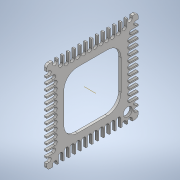
# Autodesk Inventor part: FrontPanelSquishything
Saved by Autodesk Inventor 2020 (Build 240168000, 168)
## iProperties
Created: 2019-07-06
Part Number: FrontPanelSquishything
Material: Generic
Document SubType Name: Modeling
Designer: DDeGo
Density: 1 g/cm^3
Appearance: Default
Author: DDeGo
Autodesk Inventor part; units mm, degrees
ref_plane "YZ Plane" through (0, 0, 0) normal (1, 0, 0) x (0, 1, 0)
ref_plane "XZ Plane" through (0, 0, 0) normal (0, 1, 0) x (-1, 0, 0)
ref_plane "XY Plane" through (0, 0, 0) normal (0, 0, 1) x (1, 0, 0)
sketch "Sketch1" plane through (0, 0, 0) normal (1, 0, 0) x (0, 1, 0)
  line L0 (-78.25, 91.75) -> (78.25, 91.75) construction
  line L1 (91.75, 78.25) -> (91.75, -78.25) construction
  line L2 (78.25, -91.75) -> (-78.25, -91.75) construction
  line L3 (-91.75, -78.25) -> (-91.75, 78.25) construction
  arc A0 (91.75, 78.25) -> (78.25, 91.75) centre (78.25, 78.25) ccw construction
  arc A1 (78.25, -91.75) -> (91.75, -78.25) centre (78.25, -78.25) ccw construction
  arc A2 (-91.75, -78.25) -> (-78.25, -91.75) centre (-78.25, -78.25) ccw construction
  arc A3 (-78.25, 91.75) -> (-91.75, 78.25) centre (-78.25, 78.25) ccw construction
  line L4 (-51.75, 56.75) -> (51.75, 56.75) construction
  line L5 (56.75, 51.75) -> (56.75, -51.75) construction
  line L6 (51.75, -56.75) -> (-51.75, -56.75) construction
  line L7 (-56.75, -51.75) -> (-56.75, 51.75) construction
  arc A4 (-51.75, 56.75) -> (-56.75, 51.75) centre (-51.75, 51.75) ccw construction
  arc A5 (-56.75, -51.75) -> (-51.75, -56.75) centre (-51.75, -51.75) ccw construction
  arc A6 (51.75, -56.75) -> (56.75, -51.75) centre (51.75, -51.75) ccw construction
  arc A7 (56.75, 51.75) -> (51.75, 56.75) centre (51.75, 51.75) ccw construction
  line L8 (78.25, 83.75) -> (-78.25, 83.75)
  arc A8 (-78.25, 83.75) -> (-83.75, 78.25) centre (-78.25, 78.25) ccw
  line L9 (-83.75, 78.25) -> (-83.75, -78.25)
  arc A9 (-83.75, -78.25) -> (-78.25, -83.75) centre (-78.25, -78.25) ccw
  line L10 (-78.25, -83.75) -> (78.25, -83.75)
  arc A10 (78.25, -83.75) -> (83.75, -78.25) centre (78.25, -78.25) ccw
  line L11 (83.75, -78.25) -> (83.75, 78.25)
  arc A11 (83.75, 78.25) -> (78.25, 83.75) centre (78.25, 78.25) ccw
  line L12 (-47.7, 83.75) -> (-47.7, 68.75) construction
  line L13 (-51.75, 83.75) -> (-51.75, 68.75)
  line L14 (-43.65, 68.75) -> (-43.65, 83.75)
  arc A12 (-43.65, 83.75) -> (-51.75, 83.75) centre (-47.7, 83.75) ccw
  arc A13 (-51.75, 68.75) -> (-43.65, 68.75) centre (-47.7, 68.75) ccw
  line L15 (-33.05, 68.75) -> (-33.05, 83.75)
  line L16 (-37.1, 83.75) -> (-37.1, 68.75) construction
  arc A14 (-41.15, 68.75) -> (-33.05, 68.75) centre (-37.1, 68.75) ccw
  arc A15 (-33.05, 83.75) -> (-41.15, 83.75) centre (-37.1, 83.75) ccw
  line L17 (-41.15, 83.75) -> (-41.15, 68.75)
  line L18 (-22.45, 68.75) -> (-22.45, 83.75)
  line L19 (-26.5, 83.75) -> (-26.5, 68.75) construction
  arc A16 (-30.55, 68.75) -> (-22.45, 68.75) centre (-26.5, 68.75) ccw
  arc A17 (-22.45, 83.75) -> (-30.55, 83.75) centre (-26.5, 83.75) ccw
  line L20 (-30.55, 83.75) -> (-30.55, 68.75)
  line L21 (-11.85, 68.75) -> (-11.85, 83.75)
  line L22 (-15.9, 83.75) -> (-15.9, 68.75) construction
  arc A18 (-19.95, 68.75) -> (-11.85, 68.75) centre (-15.9, 68.75) ccw
  arc A19 (-11.85, 83.75) -> (-19.95, 83.75) centre (-15.9, 83.75) ccw
  line L23 (-19.95, 83.75) -> (-19.95, 68.75)
  line L24 (-1.25, 68.75) -> (-1.25, 83.75)
  line L25 (-5.3, 83.75) -> (-5.3, 68.75) construction
  arc A20 (-9.35, 68.75) -> (-1.25, 68.75) centre (-5.3, 68.75) ccw
  arc A21 (-1.25, 83.75) -> (-9.35, 83.75) centre (-5.3, 83.75) ccw
  line L26 (-9.35, 83.75) -> (-9.35, 68.75)
  line L27 (9.35, 68.75) -> (9.35, 83.75)
  line L28 (5.3, 83.75) -> (5.3, 68.75) construction
  arc A22 (1.25, 68.75) -> (9.35, 68.75) centre (5.3, 68.75) ccw
  arc A23 (9.35, 83.75) -> (1.25, 83.75) centre (5.3, 83.75) ccw
  line L29 (1.25, 83.75) -> (1.25, 68.75)
  line L30 (19.95, 68.75) -> (19.95, 83.75)
  line L31 (15.9, 83.75) -> (15.9, 68.75) construction
  arc A24 (11.85, 68.75) -> (19.95, 68.75) centre (15.9, 68.75) ccw
  arc A25 (19.95, 83.75) -> (11.85, 83.75) centre (15.9, 83.75) ccw
  line L32 (11.85, 83.75) -> (11.85, 68.75)
  line L33 (30.55, 68.75) -> (30.55, 83.75)
  line L34 (26.5, 83.75) -> (26.5, 68.75) construction
  arc A26 (22.45, 68.75) -> (30.55, 68.75) centre (26.5, 68.75) ccw
  arc A27 (30.55, 83.75) -> (22.45, 83.75) centre (26.5, 83.75) ccw
  line L35 (22.45, 83.75) -> (22.45, 68.75)
  line L36 (41.15, 68.75) -> (41.15, 83.75)
  line L37 (37.1, 83.75) -> (37.1, 68.75) construction
  arc A28 (33.05, 68.75) -> (41.15, 68.75) centre (37.1, 68.75) ccw
  arc A29 (41.15, 83.75) -> (33.05, 83.75) centre (37.1, 83.75) ccw
  line L38 (33.05, 83.75) -> (33.05, 68.75)
  line L39 (51.75, 68.75) -> (51.75, 83.75)
  line L40 (47.7, 83.75) -> (47.7, 68.75) construction
  arc A30 (43.65, 68.75) -> (51.75, 68.75) centre (47.7, 68.75) ccw
  arc A31 (51.75, 83.75) -> (43.65, 83.75) centre (47.7, 83.75) ccw
  line L41 (43.65, 83.75) -> (43.65, 68.75)
  line L42 (-51.75, 51.75) -> (51.75, -51.75) construction
  line L43 (-58.3, 83.75) -> (-58.3, 71.75) construction
  line L44 (-62.35, 83.75) -> (-62.35, 71.75)
  line L45 (-54.25, 71.75) -> (-54.25, 83.75)
  arc A32 (-54.25, 83.75) -> (-62.35, 83.75) centre (-58.3, 83.75) ccw
  arc A33 (-62.35, 71.75) -> (-54.25, 71.75) centre (-58.3, 71.75) ccw
  line L46 (58.3, 83.75) -> (58.3, 71.75) construction
  line L47 (54.25, 83.75) -> (54.25, 71.75)
  line L48 (62.35, 71.75) -> (62.35, 83.75)
  arc A34 (62.35, 83.75) -> (54.25, 83.75) centre (58.3, 83.75) ccw
  arc A35 (54.25, 71.75) -> (62.35, 71.75) centre (58.3, 71.75) ccw
  line L49 (-68.9, 83.75) -> (-68.9, 79.75) construction
  line L50 (-72.95, 83.75) -> (-72.95, 79.75)
  line L51 (-64.85, 79.75) -> (-64.85, 83.75)
  arc A36 (-64.85, 83.75) -> (-72.95, 83.75) centre (-68.9, 83.75) ccw
  arc A37 (-72.95, 79.75) -> (-64.85, 79.75) centre (-68.9, 79.75) ccw
  line L52 (68.9, 83.75) -> (68.9, 79.75) construction
  line L53 (64.85, 83.75) -> (64.85, 79.75)
  line L54 (72.95, 79.75) -> (72.95, 83.75)
  arc A38 (72.95, 83.75) -> (64.85, 83.75) centre (68.9, 83.75) ccw
  arc A39 (64.85, 79.75) -> (72.95, 79.75) centre (68.9, 79.75) ccw
  point P0 (-47.7, 76.25)
  point P1 (-37.1, 76.25)
  point P2 (-26.5, 76.25)
  point P3 (-15.9, 76.25)
  point P4 (-5.3, 76.25)
  point P5 (5.3, 76.25)
  point P6 (15.9, 76.25)
  point P7 (26.5, 76.25)
  point P8 (37.1, 76.25)
  point P9 (47.7, 76.25)
  point P10 (0, 0)
  point P11 (-58.3, 77.75)
  point P12 (58.3, 77.75)
  point P13 (-68.9, 81.75)
  point P14 (68.9, 81.75)
  dimension "d0" = 13.5
  dimension "d1" = 183.5
  dimension "d2" = 183.5
  dimension "d15" = 35
  dimension "d16" = 35
  dimension "d17" = 35
  dimension "d18" = 35
  dimension "d19" = 5
  dimension "d20" = 8
  dimension "d21" = 15
  dimension "d25" = 10.6
  dimension "d30" = 32
  dimension "d38" = 32
  dimension "d40" = 10.6
  dimension "d41" = 12
  dimension "d42" = 10.6
  dimension "d63" = 4
  dimension "d64" = 4
  dimension "d65" = 10.6
  dimension "d66" = 10.6
  dimension "d67" = 2.5
  constraints: 138 end point, 80 point on circle, 40 centre point, 36 tangent, 12 parallel, 10 equal radius, 8 perpendicular, 6 midpoint, 5 point on line, 3 horizontal, 116 other
  measures "d0" radius of A0
  measures "d1" distance between parallel lines of L2 L0
  measures "d2" distance between parallel lines of L1 L3
  measures "d15" distance between parallel lines of L3 L7
  measures "d16" distance between parallel lines of L0 L4
  measures "d17" distance between parallel lines of L1 L5
  measures "d18" distance between parallel lines of L2 L6
  measures "d19" radius of A4
  measures "d20" distance between parallel lines of L0 L8
  measures "d21" distance of L12.start L12.end
  measures "d25" distance of L14.start L15.start
  measures "d30" distance between parallel lines of L9 L13
  measures "d38" distance between parallel lines of L11 L39
  measures "d40" distance between parallel lines of L44 L13
  measures "d41" distance of L43.start L43.end
  measures "d42" distance between parallel lines of L48 L39
  measures "d63" distance of L49.start L49.end
  measures "d64" distance of L52.start L52.end
  measures "d65" distance between parallel lines of L48 L54
  measures "d66" distance between parallel lines of L50 L44
  measures "d67" distance between parallel lines of L17 L14
extrude "Extrusion1" add sketch "Sketch1" along normal blind 4.5 contours A11 L11 A10 L10 A9 L9 A8 L8 L50 A37 L51 L44 A33 L45 L13 A13 L14 L17 A14 L15 L20 A16 L18 L23 A18 L21 L26 A20 L24 L29 A22 L27 L32 A24 L30 L35 A26 L33 L38 A28 L36 L41 A30 L39 L47 A35 L48 L53 A39 L54 | L54 A39 L53 L8 | L48 A35 L47 L8 | L39 A30 L41 L8 | L36 A28 L38 L8 | L8 L51 A37 L50 | L33 A26 L35 L8 | L8 L45 A33 L44 | L30 A24 L32 L8 | L8 L14 A13 L13 | L27 A22 L29 L8 | L8 L15 A14 L17 | L24 A20 L26 L8 | L8 L18 A16 L20 | L21 A18 L23 L8
extrude "Extrusion2" cut sketch "Sketch1" along normal blind 10 contours L54 A39 L53 L8 | L8 A38 | L48 A35 L47 L8 | L8 A34 | L39 A30 L41 L8 | L8 A31 | L36 A28 L38 L8 | L8 A29 | A36 L8 | L8 L51 A37 L50 | L33 A26 L35 L8 | L8 A27 | A32 L8 | L8 L45 A33 L44 | L30 A24 L32 L8 | L8 A25 | A12 L8 | L8 L14 A13 L13 | L27 A22 L29 L8 | L8 A23 | A15 L8 | L8 L15 A14 L17 | L24 A20 L26 L8 | L8 A21 | A17 L8 | L8 L18 A16 L20 | L21 A18 L23 L8 | L8 A19
pattern_circular "Circular Pattern1" count 4 over 360 about axis through (-10, 0, 0) along (1, 0, 0) of "Extrusion2"
sketch "Sketch3" plane through (0, 0, 0) normal (-1, 0, 0) x (0, 0, 1)
  line L0 (-27.5, 52.5) -> (27.5, 52.5)
  line L1 (52.5, 27.5) -> (52.5, -27.5)
  line L2 (27.5, -52.5) -> (-27.5, -52.5)
  line L3 (-52.5, -27.5) -> (-52.5, 27.5)
  line L4 (-52.5, 52.5) -> (52.5, -52.5) construction
  line L5 (52.5, 52.5) -> (-52.5, -52.5) construction
  arc A0 (52.5, 27.5) -> (27.5, 52.5) centre (27.5, 27.5) ccw
  arc A1 (-27.5, 52.5) -> (-52.5, 27.5) centre (-27.5, 27.5) ccw
  arc A2 (-52.5, -27.5) -> (-27.5, -52.5) centre (-27.5, -27.5) ccw
  arc A3 (27.5, -52.5) -> (52.5, -27.5) centre (27.5, -27.5) ccw
  point P0 (0, 0)
  dimension "d51" = 25
  dimension "d52" = 105
  dimension "d53" = 105
  constraints: 12 end point, 8 point on circle, 8 point on line, 8 tangent, 4 centre point, 3 equal radius, 2 midpoint, 2 parallel, 1 horizontal, 1 perpendicular
  measures "d51" radius of A0
  measures "d52" distance between parallel lines of L2 L0
  measures "d53" distance between parallel lines of L1 L3
extrude "Extrusion4" cut sketch "Sketch3" against normal blind 10
sketch "Sketch4" plane through (4.5, 0, 0) normal (1, 0, 0) x (0, 0, -1)
  line L0 (83.75, 51.75) -> (83.75, 54.25) construction
  line L1 (83.75, 62.35) -> (83.75, 64.85) construction
  line L2 (83.75, 54.25) -> (83.75, 62.35) construction
  line L3 (64.85, 83.75) -> (62.35, 83.75) construction
  line L4 (54.25, 83.75) -> (51.75, 83.75) construction
  line L5 (62.35, 83.75) -> (54.25, 83.75) construction
  line L6 (83.75, 62.35) -> (71.75, 62.35) construction
  arc A0 (79.75, 62.35) -> (79.75, 54.25) centre (79.75, 58.3) ccw
  line L7 (54.25, 71.75) -> (54.25, 83.75) construction
  line L8 (62.35, 83.75) -> (62.35, 71.75) construction
  arc A1 (54.25, 79.75) -> (62.35, 79.75) centre (58.3, 79.75) ccw
  line L9 (79.75, 62.35) -> (83.75, 62.35) construction
  line L10 (71.75, 54.25) -> (83.75, 54.25) construction
  line L11 (79.75, 54.25) -> (83.75, 54.25) construction
  line L12 (62.35, 83.75) -> (62.35, 79.75) construction
  line L13 (54.25, 79.75) -> (54.25, 83.75) construction
  line L14 (54.25, 79.75) -> (62.35, 79.75) construction
  line L15 (64.85, 79.75) -> (64.85, 83.75) projected
  line L16 (62.35, 79.75) -> (64.85, 79.75) construction
  arc A2 (79.75, 72.95) -> (79.75, 64.85) centre (79.75, 68.9) ccw projected
  line L17 (79.75, 64.85) -> (79.75, 62.35) construction
  line L18 (79.75, 62.35) -> (79.75, 54.25) construction
  line L19 (71.75, 62.35) -> (83.75, 62.35) construction
  line L20 (54.25, 79.75) -> (54.25, 54.25)
  line L21 (54.25, 54.25) -> (79.75, 54.25)
  line L22 (79.75, 62.35) -> (62.35, 62.35)
  line L23 (62.35, 79.75) -> (62.35, 62.35)
  point P0 (0, 0)
  constraints: 28 end point, 6 collinear, 6 point on line, 5 tangent, 4 point on circle, 2 centre point, 2 horizontal, 2 perpendicular, 2 vertical
extrude "Extrusion5" add sketch "Sketch4" against normal up to surface (4.5 mm away)
sketch "Sketch5" plane through (4.5, 0, 0) normal (1, 0, 0) x (0, 0, -1)
  circle A0 centre (64.75, 64.75) radius 8.1
  line L0 (78.25, 83.75) -> (51.75, 83.75) projected
  line L1 (83.75, 51.75) -> (83.75, 78.25) projected
  point P0 (0, 0)
  dimension "d58" = 19
  dimension "d59" = 19
  dimension "d60" = 16.2
  constraints: 1 centre point
  measures "d58" distance from line of L0 A0.centre
  measures "d59" distance from line of L1 A0.centre
  measures "d60" diameter of A0
extrude "Extrusion6" cut sketch "Sketch5" against normal blind 10
equation "\"d2\" = d1"
equation "\"d16\" = d15"
equation "\"d17\" = d15"
equation "\"d18\" = d15"
equation "\"d38\" = d30"
equation "\"d40\" = d25"
equation "\"d42\" = d25"
equation "\"d64\" = d63"
equation "\"d65\" = d25"
equation "\"d66\" = d25"
equation "\"d53\" = d52"
body "Solid1"
